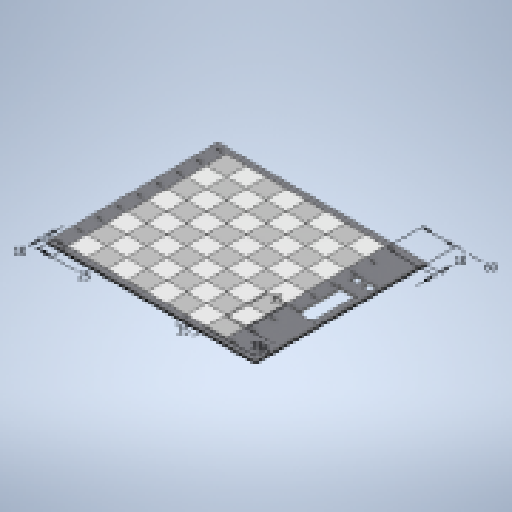
# Autodesk Inventor part: Board
Saved by Autodesk Inventor 2024 (Build 280153000, 153)
## iProperties
Created: 2023-07-19
Part Number: Board
Material: Generic
Document SubType Name: Modeling
Designer: Bruno
Density: 1 g/cm^3
Appearance: Black Tile Material
Author: Bruno
Autodesk Inventor part; units mm, degrees
ref_plane "YZ Plane" through (0, 0, 0) normal (1, 0, 0) x (0, 1, 0)
ref_plane "XZ Plane" through (0, 0, 0) normal (0, 1, 0) x (-1, 0, 0)
ref_plane "XY Plane" through (0, 0, 0) normal (0, 0, 1) x (1, 0, 0)
sketch "Sketch1" plane through (0, 0, 0) normal (0, 1, 0) x (-1, 0, 0)
  line L0 (35, 0) -> (0, 0)
  line L1 (0, 0) -> (0, -35)
  line L2 (0, -35) -> (35, -35)
  line L3 (35, -35) -> (35, 0)
  line L4 (70, 0) -> (35, 0)
  line L5 (35, 0) -> (35, -35)
  line L6 (35, -35) -> (70, -35)
  line L7 (70, -35) -> (70, 0)
  line L8 (105, 0) -> (70, 0)
  line L9 (70, 0) -> (70, -35)
  line L10 (70, -35) -> (105, -35)
  line L11 (105, -35) -> (105, 0)
  line L12 (140, 0) -> (105, 0)
  line L13 (105, 0) -> (105, -35)
  line L14 (105, -35) -> (140, -35)
  line L15 (140, -35) -> (140, 0)
  line L16 (175, 0) -> (140, 0)
  line L17 (140, 0) -> (140, -35)
  line L18 (140, -35) -> (175, -35)
  line L19 (175, -35) -> (175, 0)
  line L20 (210, 0) -> (175, 0)
  line L21 (175, 0) -> (175, -35)
  line L22 (175, -35) -> (210, -35)
  line L23 (210, -35) -> (210, 0)
  line L24 (245, 0) -> (210, 0)
  line L25 (210, 0) -> (210, -35)
  line L26 (210, -35) -> (245, -35)
  line L27 (245, -35) -> (245, 0)
  line L28 (280, 0) -> (245, 0)
  line L29 (245, 0) -> (245, -35)
  line L30 (245, -35) -> (280, -35)
  line L31 (280, -35) -> (280, 0)
  line L32 (35, -35) -> (0, -35)
  line L33 (0, -35) -> (0, -70)
  line L34 (0, -70) -> (35, -70)
  line L35 (35, -70) -> (35, -35)
  line L36 (70, -35) -> (35, -35)
  line L37 (35, -35) -> (35, -70)
  line L38 (35, -70) -> (70, -70)
  line L39 (70, -70) -> (70, -35)
  line L40 (105, -35) -> (70, -35)
  line L41 (70, -35) -> (70, -70)
  line L42 (70, -70) -> (105, -70)
  line L43 (105, -70) -> (105, -35)
  line L44 (140, -35) -> (105, -35)
  line L45 (105, -35) -> (105, -70)
  line L46 (105, -70) -> (140, -70)
  line L47 (140, -70) -> (140, -35)
  line L48 (175, -35) -> (140, -35)
  line L49 (140, -35) -> (140, -70)
  line L50 (140, -70) -> (175, -70)
  line L51 (175, -70) -> (175, -35)
  line L52 (210, -35) -> (175, -35)
  line L53 (175, -35) -> (175, -70)
  line L54 (175, -70) -> (210, -70)
  line L55 (210, -70) -> (210, -35)
  line L56 (245, -35) -> (210, -35)
  line L57 (210, -35) -> (210, -70)
  line L58 (210, -70) -> (245, -70)
  line L59 (245, -70) -> (245, -35)
  line L60 (280, -35) -> (245, -35)
  line L61 (245, -35) -> (245, -70)
  line L62 (245, -70) -> (280, -70)
  line L63 (280, -70) -> (280, -35)
  line L64 (35, -70) -> (0, -70)
  line L65 (0, -70) -> (0, -105)
  line L66 (0, -105) -> (35, -105)
  line L67 (35, -105) -> (35, -70)
  line L68 (70, -70) -> (35, -70)
  line L69 (35, -70) -> (35, -105)
  line L70 (35, -105) -> (70, -105)
  line L71 (70, -105) -> (70, -70)
  line L72 (105, -70) -> (70, -70)
  line L73 (70, -70) -> (70, -105)
  line L74 (70, -105) -> (105, -105)
  line L75 (105, -105) -> (105, -70)
  line L76 (140, -70) -> (105, -70)
  line L77 (105, -70) -> (105, -105)
  line L78 (105, -105) -> (140, -105)
  line L79 (140, -105) -> (140, -70)
  line L80 (175, -70) -> (140, -70)
  line L81 (140, -70) -> (140, -105)
  line L82 (140, -105) -> (175, -105)
  line L83 (175, -105) -> (175, -70)
  line L84 (210, -70) -> (175, -70)
  line L85 (175, -70) -> (175, -105)
  line L86 (175, -105) -> (210, -105)
  line L87 (210, -105) -> (210, -70)
  line L88 (245, -70) -> (210, -70)
  line L89 (210, -70) -> (210, -105)
  line L90 (210, -105) -> (245, -105)
  line L91 (245, -105) -> (245, -70)
  line L92 (280, -70) -> (245, -70)
  line L93 (245, -70) -> (245, -105)
  line L94 (245, -105) -> (280, -105)
  line L95 (280, -105) -> (280, -70)
  line L96 (35, -105) -> (0, -105)
  line L97 (0, -105) -> (0, -140)
  line L98 (0, -140) -> (35, -140)
  line L99 (35, -140) -> (35, -105)
  line L100 (70, -105) -> (35, -105)
  line L101 (35, -105) -> (35, -140)
  line L102 (35, -140) -> (70, -140)
  line L103 (70, -140) -> (70, -105)
  line L104 (105, -105) -> (70, -105)
  line L105 (70, -105) -> (70, -140)
  line L106 (70, -140) -> (105, -140)
  line L107 (105, -140) -> (105, -105)
  line L108 (140, -105) -> (105, -105)
  line L109 (105, -105) -> (105, -140)
  line L110 (105, -140) -> (140, -140)
  line L111 (140, -140) -> (140, -105)
  line L112 (175, -105) -> (140, -105)
  line L113 (140, -105) -> (140, -140)
  line L114 (140, -140) -> (175, -140)
  line L115 (175, -140) -> (175, -105)
  line L116 (210, -105) -> (175, -105)
  line L117 (175, -105) -> (175, -140)
  line L118 (175, -140) -> (210, -140)
  line L119 (210, -140) -> (210, -105)
  line L120 (245, -105) -> (210, -105)
  line L121 (210, -105) -> (210, -140)
  line L122 (210, -140) -> (245, -140)
  line L123 (245, -140) -> (245, -105)
  line L124 (280, -105) -> (245, -105)
  line L125 (245, -105) -> (245, -140)
  line L126 (245, -140) -> (280, -140)
  line L127 (280, -140) -> (280, -105)
  line L128 (35, -140) -> (0, -140)
  line L129 (0, -140) -> (0, -175)
  line L130 (0, -175) -> (35, -175)
  line L131 (35, -175) -> (35, -140)
  line L132 (70, -140) -> (35, -140)
  line L133 (35, -140) -> (35, -175)
  line L134 (35, -175) -> (70, -175)
  line L135 (70, -175) -> (70, -140)
  line L136 (105, -140) -> (70, -140)
  line L137 (70, -140) -> (70, -175)
  line L138 (70, -175) -> (105, -175)
  line L139 (105, -175) -> (105, -140)
  line L140 (140, -140) -> (105, -140)
  line L141 (105, -140) -> (105, -175)
  line L142 (105, -175) -> (140, -175)
  line L143 (140, -175) -> (140, -140)
  line L144 (175, -140) -> (140, -140)
  line L145 (140, -140) -> (140, -175)
  line L146 (140, -175) -> (175, -175)
  line L147 (175, -175) -> (175, -140)
  line L148 (210, -140) -> (175, -140)
  line L149 (175, -140) -> (175, -175)
  line L150 (175, -175) -> (210, -175)
  line L151 (210, -175) -> (210, -140)
  line L152 (245, -140) -> (210, -140)
  line L153 (210, -140) -> (210, -175)
  line L154 (210, -175) -> (245, -175)
  line L155 (245, -175) -> (245, -140)
  line L156 (280, -140) -> (245, -140)
  line L157 (245, -140) -> (245, -175)
  line L158 (245, -175) -> (280, -175)
  line L159 (280, -175) -> (280, -140)
  line L160 (35, -175) -> (0, -175)
  line L161 (0, -175) -> (0, -210)
  line L162 (0, -210) -> (35, -210)
  line L163 (35, -210) -> (35, -175)
  line L164 (70, -175) -> (35, -175)
  line L165 (35, -175) -> (35, -210)
  line L166 (35, -210) -> (70, -210)
  line L167 (70, -210) -> (70, -175)
  line L168 (105, -175) -> (70, -175)
  line L169 (70, -175) -> (70, -210)
  line L170 (70, -210) -> (105, -210)
  line L171 (105, -210) -> (105, -175)
  line L172 (140, -175) -> (105, -175)
  line L173 (105, -175) -> (105, -210)
  line L174 (105, -210) -> (140, -210)
  line L175 (140, -210) -> (140, -175)
  line L176 (175, -175) -> (140, -175)
  line L177 (140, -175) -> (140, -210)
  line L178 (140, -210) -> (175, -210)
  line L179 (175, -210) -> (175, -175)
  line L180 (210, -175) -> (175, -175)
  line L181 (175, -175) -> (175, -210)
  line L182 (175, -210) -> (210, -210)
  line L183 (210, -210) -> (210, -175)
  line L184 (245, -175) -> (210, -175)
  line L185 (210, -175) -> (210, -210)
  line L186 (210, -210) -> (245, -210)
  line L187 (245, -210) -> (245, -175)
  line L188 (280, -175) -> (245, -175)
  line L189 (245, -175) -> (245, -210)
  line L190 (245, -210) -> (280, -210)
  line L191 (280, -210) -> (280, -175)
  line L192 (35, -210) -> (0, -210)
  line L193 (0, -210) -> (0, -245)
  line L194 (0, -245) -> (35, -245)
  line L195 (35, -245) -> (35, -210)
  line L196 (70, -210) -> (35, -210)
  line L197 (35, -210) -> (35, -245)
  line L198 (35, -245) -> (70, -245)
  line L199 (70, -245) -> (70, -210)
  line L200 (105, -210) -> (70, -210)
  line L201 (70, -210) -> (70, -245)
  line L202 (70, -245) -> (105, -245)
  line L203 (105, -245) -> (105, -210)
  line L204 (140, -210) -> (105, -210)
  line L205 (105, -210) -> (105, -245)
  line L206 (105, -245) -> (140, -245)
  line L207 (140, -245) -> (140, -210)
  line L208 (175, -210) -> (140, -210)
  line L209 (140, -210) -> (140, -245)
  line L210 (140, -245) -> (175, -245)
  line L211 (175, -245) -> (175, -210)
  line L212 (210, -210) -> (175, -210)
  line L213 (175, -210) -> (175, -245)
  line L214 (175, -245) -> (210, -245)
  line L215 (210, -245) -> (210, -210)
  line L216 (245, -210) -> (210, -210)
  line L217 (210, -210) -> (210, -245)
  line L218 (210, -245) -> (245, -245)
  line L219 (245, -245) -> (245, -210)
  line L220 (280, -210) -> (245, -210)
  line L221 (245, -210) -> (245, -245)
  line L222 (245, -245) -> (280, -245)
  line L223 (280, -245) -> (280, -210)
  line L224 (35, -245) -> (0, -245)
  line L225 (0, -245) -> (0, -280)
  line L226 (0, -280) -> (35, -280)
  line L227 (35, -280) -> (35, -245)
  line L228 (70, -245) -> (35, -245)
  line L229 (35, -245) -> (35, -280)
  line L230 (35, -280) -> (70, -280)
  line L231 (70, -280) -> (70, -245)
  line L232 (105, -245) -> (70, -245)
  line L233 (70, -245) -> (70, -280)
  line L234 (70, -280) -> (105, -280)
  line L235 (105, -280) -> (105, -245)
  line L236 (140, -245) -> (105, -245)
  line L237 (105, -245) -> (105, -280)
  line L238 (105, -280) -> (140, -280)
  line L239 (140, -280) -> (140, -245)
  line L240 (175, -245) -> (140, -245)
  line L241 (140, -245) -> (140, -280)
  line L242 (140, -280) -> (175, -280)
  line L243 (175, -280) -> (175, -245)
  line L244 (210, -245) -> (175, -245)
  line L245 (175, -245) -> (175, -280)
  line L246 (175, -280) -> (210, -280)
  line L247 (210, -280) -> (210, -245)
  line L248 (245, -245) -> (210, -245)
  line L249 (210, -245) -> (210, -280)
  line L250 (210, -280) -> (245, -280)
  line L251 (245, -280) -> (245, -245)
  line L252 (280, -245) -> (245, -245)
  line L253 (245, -245) -> (245, -280)
  line L254 (245, -280) -> (280, -280)
  line L255 (280, -280) -> (280, -245)
  line L256 (-60, 10) -> (305, 10)
  line L257 (305, 10) -> (305, -290)
  line L258 (305, -290) -> (-60, -290)
  line L259 (-60, -290) -> (-60, 10)
  point P0 (35, -70)
  point P1 (35, -70)
  point P2 (245, -105)
  point P3 (245, -105)
  point P4 (245, 0)
  point P5 (245, -35)
  point P6 (245, -35)
  point P7 (175, 0)
  point P8 (175, -35)
  point P9 (175, -35)
  point P10 (210, -35)
  point P11 (210, -35)
  point P12 (105, 0)
  point P13 (140, -35)
  point P14 (35, 0)
  point P15 (70, -35)
  point P16 (70, -35)
  point P17 (175, -70)
  point P18 (175, -70)
  point P19 (280, -35)
  point P20 (210, 0)
  point P21 (140, 0)
  point P22 (70, 0)
  dimension "d0" = 35
  dimension "d1" = 35
  dimension "d4" = 35
  dimension "d7" = 35
  dimension "d10" = 10
  dimension "d12" = 10
  dimension "d13" = 25
  dimension "d14" = 60
  constraints: 520 end point, 4 parallel, 3 horizontal, 2 collinear, 2 perpendicular, 1 coincident, 1 vertical, 502 other
  measures "d0" distance between parallel lines of L1 L3
  measures "d1" distance of L2.end L0.start
  measures "d4" distance of L0.start L4.start
  measures "d7" distance of L0.start L32.start
  measures "d10" distance between parallel lines of L258 L226
  measures "d12" distance between parallel lines of L28 L256
  measures "d13" distance between parallel lines of L257 L31
  measures "d14" distance between parallel lines of L225 L259
extrude "WhiteTiles" add sketch "Sketch1" along normal blind 3.1 contours L3 L2 L1 L0 | L6 L39 L38 L35 | L8 L11 L10 L7 | L67 L66 L65 L34 | L14 L47 L46 L43 | L42 L75 L74 L71 | L70 L103 L102 L99 | L16 L19 L18 L15 | L131 L130 L129 L98 | L22 L55 L54 L51 | L50 L83 L82 L79 | L78 L111 L110 L107 | L106 L139 L138 L135 | L134 L167 L166 L163 | L24 L27 L26 L23 | L195 L194 L193 L162 | L30 L63 L62 L59 | L58 L91 L90 L87 | L86 L119 L118 L115 | L114 L147 L146 L143 | L142 L175 L174 L171 | L170 L203 L202 L199 | L198 L231 L230 L227 | L94 L127 L126 L123 | L122 L155 L154 L151 | L150 L183 L182 L179 | L178 L211 L210 L207 | L206 L239 L238 L235 | L158 L191 L190 L187 | L186 L219 L218 L215 | L214 L247 L246 L243 | L222 L255 L254 L251
extrude "BlackTiles" add sketch "Sketch1" along normal blind 3 contours L4 L7 L6 L3 | L35 L34 L33 L2 | L10 L43 L42 L39 | L38 L71 L70 L67 | L12 L15 L14 L11 | L99 L98 L97 L66 | L18 L51 L50 L47 | L46 L79 L78 L75 | L74 L107 L106 L103 | L102 L135 L134 L131 | L20 L23 L22 L19 | L163 L162 L161 L130 | L26 L59 L58 L55 | L54 L87 L86 L83 | L82 L115 L114 L111 | L110 L143 L142 L139 | L138 L171 L170 L167 | L166 L199 L198 L195 | L28 L31 L30 L27 | L227 L226 L225 L194 | L62 L95 L94 L91 | L90 L123 L122 L119 | L118 L151 L150 L147 | L146 L179 L178 L175 | L174 L207 L206 L203 | L202 L235 L234 L231 | L126 L159 L158 L155 | L154 L187 L186 L183 | L182 L215 L214 L211 | L210 L243 L242 L239 | L190 L223 L222 L219 | L218 L251 L250 L247
extrude "Border" add sketch "Sketch1" along normal blind 2.9
sketch "Sketch2" plane through (0, 2.9, 0) normal (0, 1, 0) x (1, 0, 0)
  line L0 (60, 290) -> (60, -10) projected
  line L1 (60, -10) -> (-305, -10) projected
  line L2 (-305, -10) -> (-305, 290) projected
  line L3 (-305, 290) -> (60, 290) projected
  line L4 (-280, 0) -> (0, 0) projected
  line L5 (0, 0) -> (0, 280) projected
  line L6 (0, 280) -> (-280, 280) projected
  line L7 (-280, 280) -> (-280, 0) projected
  line L8 (-296.55, 68.5) -> (-288.55, 68.5) projected
  line L9 (-288.55, 68.5) -> (-288.55, 71.5) projected
  line L10 (-296.55, 71.5) -> (-288.55, 71.5) projected
  line L11 (-296.55, 68.5) -> (-296.55, 71.5) projected
  line L12 (-296.55, 103.5) -> (-288.55, 103.5) projected
  line L13 (-288.55, 103.5) -> (-288.55, 106.5) projected
  line L14 (-296.55, 106.5) -> (-288.55, 106.5) projected
  line L15 (-296.55, 103.5) -> (-296.55, 106.5) projected
  line L16 (-296.55, 138.5) -> (-288.55, 138.5) projected
  line L17 (-288.55, 138.5) -> (-288.55, 141.5) projected
  line L18 (-296.55, 141.5) -> (-288.55, 141.5) projected
  line L19 (-296.55, 138.5) -> (-296.55, 141.5) projected
  line L20 (-296.55, 173.5) -> (-288.55, 173.5) projected
  line L21 (-288.55, 173.5) -> (-288.55, 176.5) projected
  line L22 (-296.55, 176.5) -> (-288.55, 176.5) projected
  line L23 (-296.55, 173.5) -> (-296.55, 176.5) projected
  line L24 (-296.55, 208.5) -> (-288.55, 208.5) projected
  line L25 (-288.55, 208.5) -> (-288.55, 211.5) projected
  line L26 (-296.55, 211.5) -> (-288.55, 211.5) projected
  line L27 (-296.55, 208.5) -> (-296.55, 211.5) projected
  line L28 (-296.55, 243.5) -> (-288.55, 243.5) projected
  line L29 (-288.55, 243.5) -> (-288.55, 246.5) projected
  line L30 (-296.55, 246.5) -> (-288.55, 246.5) projected
  line L31 (-296.55, 243.5) -> (-296.55, 246.5) projected
  line L32 (-296.55, 278.5) -> (-288.55, 278.5) projected
  line L33 (-288.55, 278.5) -> (-288.55, 281.5) projected
  line L34 (-296.55, 281.5) -> (-288.55, 281.5) projected
  line L35 (-296.55, 278.5) -> (-296.55, 281.5) projected
  line L36 (8.55, 278.5) -> (16.55, 278.5) projected
  line L37 (16.55, 278.5) -> (16.55, 281.5) projected
  line L38 (8.55, 281.5) -> (16.55, 281.5) projected
  line L39 (8.55, 278.5) -> (8.55, 281.5) projected
  line L40 (8.55, 243.5) -> (16.55, 243.5) projected
  line L41 (16.55, 243.5) -> (16.55, 246.5) projected
  line L42 (8.55, 246.5) -> (16.55, 246.5) projected
  line L43 (8.55, 243.5) -> (8.55, 246.5) projected
  line L44 (8.55, 103.5) -> (16.55, 103.5) projected
  line L45 (16.55, 103.5) -> (16.55, 106.5) projected
  line L46 (8.55, 106.5) -> (16.55, 106.5) projected
  line L47 (8.55, 103.5) -> (8.55, 106.5) projected
  line L48 (8.55, 138.5) -> (16.55, 138.5) projected
  line L49 (16.55, 138.5) -> (16.55, 141.5) projected
  line L50 (8.55, 141.5) -> (16.55, 141.5) projected
  line L51 (8.55, 138.5) -> (8.55, 141.5) projected
  line L52 (8.55, 208.5) -> (16.55, 208.5) projected
  line L53 (16.55, 208.5) -> (16.55, 211.5) projected
  line L54 (8.55, 211.5) -> (16.55, 211.5) projected
  line L55 (8.55, 208.5) -> (8.55, 211.5) projected
  line L56 (8.55, 173.5) -> (16.55, 173.5) projected
  line L57 (16.55, 173.5) -> (16.55, 176.5) projected
  line L58 (8.55, 176.5) -> (16.55, 176.5) projected
  line L59 (8.55, 173.5) -> (8.55, 176.5) projected
  line L60 (8.55, -1.5) -> (16.55, -1.5) projected
  line L61 (16.55, -1.5) -> (16.55, 1.5) projected
  line L62 (8.55, 1.5) -> (16.55, 1.5) projected
  line L63 (8.55, -1.5) -> (8.55, 1.5) projected
  line L64 (8.55, 33.5) -> (16.55, 33.5) projected
  line L65 (16.55, 33.5) -> (16.55, 36.5) projected
  line L66 (8.55, 36.5) -> (16.55, 36.5) projected
  line L67 (8.55, 33.5) -> (8.55, 36.5) projected
  line L68 (8.55, 68.5) -> (16.55, 68.5) projected
  line L69 (16.55, 68.5) -> (16.55, 71.5) projected
  line L70 (8.55, 71.5) -> (16.55, 71.5) projected
  line L71 (8.55, 68.5) -> (8.55, 71.5) projected
  line L72 (-296.55, -1.5) -> (-288.55, -1.5) projected
  line L73 (-288.55, -1.5) -> (-288.55, 1.5) projected
  line L74 (-296.55, 1.5) -> (-288.55, 1.5) projected
  line L75 (-296.55, -1.5) -> (-296.55, 1.5) projected
  line L76 (-296.55, 33.5) -> (-288.55, 33.5) projected
  line L77 (-288.55, 33.5) -> (-288.55, 36.5) projected
  line L78 (-296.55, 36.5) -> (-288.55, 36.5) projected
  line L79 (-296.55, 33.5) -> (-296.55, 36.5) projected
extrude "SeperatorPinSlots" cut sketch "Sketch2" against normal up to surface (2.9 mm away) contours L11 L10 L9 L8 | L15 L14 L13 L12 | L19 L18 L17 L16 | L23 L22 L21 L20 | L27 L26 L25 L24 | L31 L30 L29 L28 | L35 L34 L33 L32 | L39 L38 L37 L36 | L43 L42 L41 L40 | L47 L46 L45 L44 | L51 L50 L49 L48 | L55 L54 L53 L52 | L59 L58 L57 L56 | L63 L62 L61 L60 | L67 L66 L65 L64 | L71 L70 L69 L68 | L75 L74 L73 L72 | L79 L78 L77 L76
sketch "Sketch3" plane through (0, 2.9, 0) normal (0, 1, 0) x (1, 0, 0)
  line L0 (24, 43) -> (24, 116)
  line L1 (24, 116) -> (50, 116)
  line L2 (50, 116) -> (50, 43)
  line L3 (37, 40) -> (37, -10) construction
  line L4 (-305, -10) -> (60, -10) projected
  line L5 (60, 290) -> (-305, 290) projected
  line L6 (60, -10) -> (60, 290) projected
  circle A0 centre (21.5, 117) radius 1.5
  circle A1 centre (52.5, 117) radius 1.5
  circle A2 centre (52.5, 42) radius 1.5
  circle A3 centre (21.5, 42) radius 1.5
  line L7 (52.5, 42) -> (52.5, 79.5) construction
  line L8 (21.5, 42) -> (37, 42) construction
  line L9 (37, 42) -> (52.5, 42) construction
  line L10 (50, 43) -> (45, 43)
  line L11 (45, 43) -> (42, 40)
  line L12 (42, 40) -> (32, 40)
  line L13 (32, 40) -> (29, 43)
  line L14 (29, 43) -> (24, 43)
  line L15 (60, -10) -> (60, 290) projected
  line L16 (41.5, 164) -> (55, 164)
  line L17 (55, 164) -> (55, 177.5)
  line L18 (55, 177.5) -> (41.5, 177.5)
  line L19 (41.5, 177.5) -> (41.5, 164)
  line L20 (20, 164) -> (33.5, 164)
  line L21 (33.5, 164) -> (33.5, 177.5)
  line L22 (33.5, 177.5) -> (20, 177.5)
  line L23 (20, 177.5) -> (20, 164)
  circle A4 centre (-122.5, 265) radius 12.5
  line L24 (60, 265) -> (-305, 265) construction
  line L25 (-305, 290) -> (-305, -10) projected
  circle A5 centre (37, 140) radius 12.5
  point P0 (0, 0)
  point P1 (26.5, 43)
  point P2 (-122.5, 290)
  dimension "d23" = 73
  dimension "d24" = 26
  dimension "d26" = 3
  dimension "d27" = 3
  dimension "d28" = 3
  dimension "d29" = 3
  dimension "d30" = 31
  dimension "d31" = 75
  dimension "d34" = 135
  dimension "d35" = 135
  dimension "d36" = 10
  dimension "d37" = 3
  dimension "d41" = 13.5
  dimension "d42" = 13.5
  dimension "d43" = 8
  dimension "d44" = 5
  dimension "d46" = 25
  dimension "d47" = 25
  dimension "d48" = 50
  dimension "d49" = 1
  dimension "d50" = 10
  dimension "d51" = 25
  dimension "d52" = 24
  dimension "d53" = 24
  constraints: 43 end point, 6 centre point, 6 horizontal, 6 parallel, 5 equal length, 4 midpoint, 4 point on line, 3 horizontal alignment, 3 vertical alignment, 2 perpendicular, 2 vertical, 1 coincident, 1 collinear
  measures "d23" distance of L1.end L2.end
  measures "d24" distance of L0.end L1.end
  measures "d26" diameter of A0
  measures "d27" diameter of A1
  measures "d28" diameter of A2
  measures "d29" diameter of A3
  measures "d30" distance of L8.start L7.start
  measures "d31" distance of A1.centre L7.start
  measures "d34" angle of L11 L10
  measures "d35" angle of L12 L13
  measures "d36" distance of L11.end L12.end
  measures "d37" distance from line of point (26.5, 43) L12
  measures "d41" distance of L16.end L17.end
  measures "d42" distance of L20.end L21.end
  measures "d43" distance between parallel lines of L19 L21
  measures "d44" distance between parallel lines of L6 L17
  measures "d46" diameter of A4
  measures "d47" distance of point (-122.5, 290) point (-122.5, 265)
  measures "d48" distance of L3.start L3.end
  measures "d49" distance from line of L1 A0.centre
  measures "d50" distance between parallel lines of L6 L2
  measures "d51" diameter of A5
  measures "d52" distance from line of L1 A5.centre
  measures "d53" vertical distance of L16.end A5.centre
extrude "Controls" cut sketch "Sketch3" against normal up to surface (2.9 mm away) contours L0 L1 L2 L10 L11 L12 L13 L14 | A0 | A1 | A2 | A3 | L19 L18 L17 L16 | L23 L22 L21 L20 | A5
body "Solid1"
